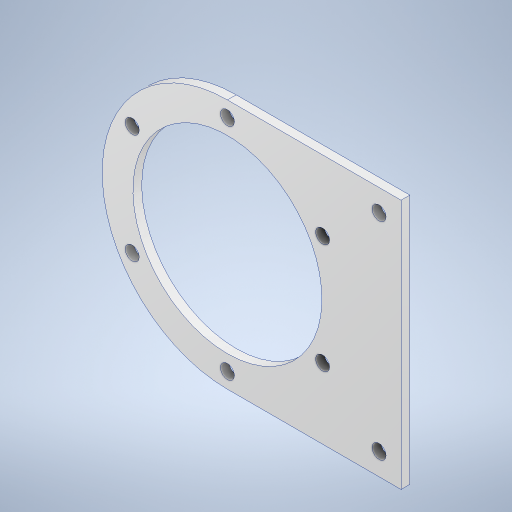
# Autodesk Inventor part: link4_plate3
Saved by Autodesk Inventor 2024 (Build 280153000, 153)
## iProperties
Created: 2024-12-13
Part Number: link4_plate3
Material: アルミニウム 6061
Document SubType Name: Modeling
Designer: hirek
Density: 2.7 g/cm^3
Appearance: アルミニウム - フラット
Mass: 7.47273 g
Surface Area: 36.0577 cm^2
Volume: 2.76768 cm^3
Author: hirek
Autodesk Inventor part; units mm, degrees
ref_plane "YZ Plane" through (0, 0, 0) normal (1, 0, 0) x (0, 1, 0)
ref_plane "XZ Plane" through (0, 0, 0) normal (0, 1, 0) x (-1, 0, 0)
ref_plane "XY Plane" through (0, 0, 0) normal (0, 0, 1) x (1, 0, 0)
sketch "スケッチ1" plane through (0, 0, 0) normal (0, 0, 1) x (1, 0, 0)
  circle A0 centre (0, 0) radius 28.5
  line L0 (0, 28.5) -> (39.5, 28.5)
  line L1 (39.5, 28.5) -> (39.5, -28.5)
  line L2 (39.5, -28.5) -> (0, -28.5)
  line L3 (0, -28.5) -> (0, 28.5)
  circle A1 centre (0, 0) radius 21.5
  point P0 (28.5, 0)
  point P1 (0, -21.5)
  point P2 (0, 21.5)
  dimension "d0" = 57
  dimension "d23" = 43
  dimension "d24" = 39.5
  constraints: 8 end point, 2 coincident, 2 parallel, 1 centre point, 1 horizontal, 1 perpendicular, 3 other
  measures "d23" diameter of A1
  measures "d24" distance between parallel lines of L1 L3
extrude "押し出し1" add sketch "スケッチ1" along normal blind 2 contours A0 L3 A1 | A0 L0 L1 L2 | L3 A1 A0
sketch "スケッチ3" plane through (0, 0, 2) normal (0, 0, 1) x (1, 0, 0)
  circle A0 centre (0, 0) radius 25
  line L0 (39.5, 28.5) -> (0, 28.5) projected
  line L1 (34.5, 28.5) -> (34.5, -28.5)
  line L2 (0, -28.5) -> (39.5, -28.5) projected
  line L3 (39.5, -28.5) -> (39.5, 28.5) projected
  line L4 (0, 0) -> (21.6506, -12.5)
  line L5 (0, 0) -> (25, 0) construction
  point P0 (34.5, 23.5)
  point P1 (34.5, -23.5)
  point P2 (21.6506, 12.5)
  point P3 (0, 25)
  point P4 (-21.6506, 12.5)
  point P5 (-21.6506, -12.5)
  point P6 (0, -25)
  dimension "d25" = 50
  dimension "d26" = 5
  dimension "d27" = 5
  dimension "d28" = 5
  dimension "d29" = 30
  dimension "d32" = 360
  constraints: 6 end point, 4 point on line, 2 coincident, 1 equal length, 1 horizontal, 1 vertical, 10 other
  measures "d26" distance between parallel lines of L3 L1
  measures "d27" distance from line of point (34.5, 23.5) L0
  measures "d28" distance from line of L2 point (34.5, -23.5)
  measures "d29" angle of L4 L5
hole "穴2" at (34.5, 23.5, 2) at (34.5, -23.5, 2) at (21.6506, -12.5, 2) at (21.6506, 12.5, 2) at (0, 25, 2) at (-21.6506, 12.5, 2) at (-21.6506, -12.5, 2) at (0, -25, 2) direction (0, 0, -1) diameter 3.2 end through all
